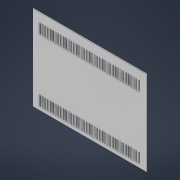
# Autodesk Inventor part: motorRAMM
Saved by Autodesk Inventor 2022 (Build 260153070, 153G)
## iProperties
Created: 2021-12-13
Part Number: motorRAMM
Material: Сталь, окрашенная, слоновая кость, матовая
Document SubType Name: Sheet Metal
Designer: A
Density: 7.85 g/cm^3
Appearance: Гладкая — черная
Mass: 360.681 g
Surface Area: 675.352 cm^2
Volume: 45.9466 cm^3
Sheet Metal Rule: По умолчанию_мм
Author: A
Autodesk Inventor part; units mm, degrees
ref_plane "YZ Plane" through (0, 0, 0) normal (1, 0, 0) x (0, 1, 0)
ref_plane "XZ Plane" through (0, 0, 0) normal (0, 1, 0) x (-1, 0, 0)
ref_plane "XY Plane" through (0, 0, 0) normal (0, 0, 1) x (1, 0, 0)
sketch "Эскиз2" plane through (0, 0, 0) normal (0, 0, 1) x (1, 0, 0)
  line L0 (6, 0) -> (6, 18) construction
  line L1 (7.5, 0) -> (7.5, 18)
  line L2 (4.5, 18) -> (4.5, 0)
  arc A0 (4.5, 0) -> (7.5, 0) centre (6, 0) ccw
  arc A1 (7.5, 18) -> (4.5, 18) centre (6, 18) ccw
  line L3 (210, -7.5) -> (-8, -7.5)
  line L4 (-8, -7.5) -> (-8, 155.5)
  line L5 (-8, 155.5) -> (210, 155.5)
  line L6 (210, 155.5) -> (210, -7.5)
  line L7 (11, 0) -> (11, 18) construction
  line L8 (12.5, 0) -> (12.5, 18)
  line L9 (9.5, 18) -> (9.5, 0)
  arc A2 (9.5, 0) -> (12.5, 0) centre (11, 0) ccw
  arc A3 (12.5, 18) -> (9.5, 18) centre (11, 18) ccw
  line L10 (16, 0) -> (16, 18) construction
  line L11 (17.5, 0) -> (17.5, 18)
  line L12 (14.5, 18) -> (14.5, 0)
  arc A4 (14.5, 0) -> (17.5, 0) centre (16, 0) ccw
  arc A5 (17.5, 18) -> (14.5, 18) centre (16, 18) ccw
  line L13 (21, 0) -> (21, 18) construction
  line L14 (22.5, 0) -> (22.5, 18)
  line L15 (19.5, 18) -> (19.5, 0)
  arc A6 (19.5, 0) -> (22.5, 0) centre (21, 0) ccw
  arc A7 (22.5, 18) -> (19.5, 18) centre (21, 18) ccw
  line L16 (26, 0) -> (26, 18) construction
  line L17 (27.5, 0) -> (27.5, 18)
  line L18 (24.5, 18) -> (24.5, 0)
  arc A8 (24.5, 0) -> (27.5, 0) centre (26, 0) ccw
  arc A9 (27.5, 18) -> (24.5, 18) centre (26, 18) ccw
  line L19 (31, 0) -> (31, 18) construction
  line L20 (32.5, 0) -> (32.5, 18)
  line L21 (29.5, 18) -> (29.5, 0)
  arc A10 (29.5, 0) -> (32.5, 0) centre (31, 0) ccw
  arc A11 (32.5, 18) -> (29.5, 18) centre (31, 18) ccw
  line L22 (36, 0) -> (36, 18) construction
  line L23 (37.5, 0) -> (37.5, 18)
  line L24 (34.5, 18) -> (34.5, 0)
  arc A12 (34.5, 0) -> (37.5, 0) centre (36, 0) ccw
  arc A13 (37.5, 18) -> (34.5, 18) centre (36, 18) ccw
  line L25 (41, 0) -> (41, 18) construction
  line L26 (42.5, 0) -> (42.5, 18)
  line L27 (39.5, 18) -> (39.5, 0)
  arc A14 (39.5, 0) -> (42.5, 0) centre (41, 0) ccw
  arc A15 (42.5, 18) -> (39.5, 18) centre (41, 18) ccw
  line L28 (46, 0) -> (46, 18) construction
  line L29 (47.5, 0) -> (47.5, 18)
  line L30 (44.5, 18) -> (44.5, 0)
  arc A16 (44.5, 0) -> (47.5, 0) centre (46, 0) ccw
  arc A17 (47.5, 18) -> (44.5, 18) centre (46, 18) ccw
  line L31 (51, 0) -> (51, 18) construction
  line L32 (52.5, 0) -> (52.5, 18)
  line L33 (49.5, 18) -> (49.5, 0)
  arc A18 (49.5, 0) -> (52.5, 0) centre (51, 0) ccw
  arc A19 (52.5, 18) -> (49.5, 18) centre (51, 18) ccw
  line L34 (56, 0) -> (56, 18) construction
  line L35 (57.5, 0) -> (57.5, 18)
  line L36 (54.5, 18) -> (54.5, 0)
  arc A20 (54.5, 0) -> (57.5, 0) centre (56, 0) ccw
  arc A21 (57.5, 18) -> (54.5, 18) centre (56, 18) ccw
  line L37 (61, 0) -> (61, 18) construction
  line L38 (62.5, 0) -> (62.5, 18)
  line L39 (59.5, 18) -> (59.5, 0)
  arc A22 (59.5, 0) -> (62.5, 0) centre (61, 0) ccw
  arc A23 (62.5, 18) -> (59.5, 18) centre (61, 18) ccw
  line L40 (66, 0) -> (66, 18) construction
  line L41 (67.5, 0) -> (67.5, 18)
  line L42 (64.5, 18) -> (64.5, 0)
  arc A24 (64.5, 0) -> (67.5, 0) centre (66, 0) ccw
  arc A25 (67.5, 18) -> (64.5, 18) centre (66, 18) ccw
  line L43 (71, 0) -> (71, 18) construction
  line L44 (72.5, 0) -> (72.5, 18)
  line L45 (69.5, 18) -> (69.5, 0)
  arc A26 (69.5, 0) -> (72.5, 0) centre (71, 0) ccw
  arc A27 (72.5, 18) -> (69.5, 18) centre (71, 18) ccw
  line L46 (76, 0) -> (76, 18) construction
  line L47 (77.5, 0) -> (77.5, 18)
  line L48 (74.5, 18) -> (74.5, 0)
  arc A28 (74.5, 0) -> (77.5, 0) centre (76, 0) ccw
  arc A29 (77.5, 18) -> (74.5, 18) centre (76, 18) ccw
  line L49 (81, 0) -> (81, 18) construction
  line L50 (82.5, 0) -> (82.5, 18)
  line L51 (79.5, 18) -> (79.5, 0)
  arc A30 (79.5, 0) -> (82.5, 0) centre (81, 0) ccw
  arc A31 (82.5, 18) -> (79.5, 18) centre (81, 18) ccw
  line L52 (86, 0) -> (86, 18) construction
  line L53 (87.5, 0) -> (87.5, 18)
  line L54 (84.5, 18) -> (84.5, 0)
  arc A32 (84.5, 0) -> (87.5, 0) centre (86, 0) ccw
  arc A33 (87.5, 18) -> (84.5, 18) centre (86, 18) ccw
  line L55 (91, 0) -> (91, 18) construction
  line L56 (92.5, 0) -> (92.5, 18)
  line L57 (89.5, 18) -> (89.5, 0)
  arc A34 (89.5, 0) -> (92.5, 0) centre (91, 0) ccw
  arc A35 (92.5, 18) -> (89.5, 18) centre (91, 18) ccw
  line L58 (96, 0) -> (96, 18) construction
  line L59 (97.5, 0) -> (97.5, 18)
  line L60 (94.5, 18) -> (94.5, 0)
  arc A36 (94.5, 0) -> (97.5, 0) centre (96, 0) ccw
  arc A37 (97.5, 18) -> (94.5, 18) centre (96, 18) ccw
  line L61 (101, 0) -> (101, 18) construction
  line L62 (102.5, 0) -> (102.5, 18)
  line L63 (99.5, 18) -> (99.5, 0)
  arc A38 (99.5, 0) -> (102.5, 0) centre (101, 0) ccw
  arc A39 (102.5, 18) -> (99.5, 18) centre (101, 18) ccw
  line L64 (106, 0) -> (106, 18) construction
  line L65 (107.5, 0) -> (107.5, 18)
  line L66 (104.5, 18) -> (104.5, 0)
  arc A40 (104.5, 0) -> (107.5, 0) centre (106, 0) ccw
  arc A41 (107.5, 18) -> (104.5, 18) centre (106, 18) ccw
  line L67 (111, 0) -> (111, 18) construction
  line L68 (112.5, 0) -> (112.5, 18)
  line L69 (109.5, 18) -> (109.5, 0)
  arc A42 (109.5, 0) -> (112.5, 0) centre (111, 0) ccw
  arc A43 (112.5, 18) -> (109.5, 18) centre (111, 18) ccw
  line L70 (116, 0) -> (116, 18) construction
  line L71 (117.5, 0) -> (117.5, 18)
  line L72 (114.5, 18) -> (114.5, 0)
  arc A44 (114.5, 0) -> (117.5, 0) centre (116, 0) ccw
  arc A45 (117.5, 18) -> (114.5, 18) centre (116, 18) ccw
  line L73 (121, 0) -> (121, 18) construction
  line L74 (122.5, 0) -> (122.5, 18)
  line L75 (119.5, 18) -> (119.5, 0)
  arc A46 (119.5, 0) -> (122.5, 0) centre (121, 0) ccw
  arc A47 (122.5, 18) -> (119.5, 18) centre (121, 18) ccw
  line L76 (126, 0) -> (126, 18) construction
  line L77 (127.5, 0) -> (127.5, 18)
  line L78 (124.5, 18) -> (124.5, 0)
  arc A48 (124.5, 0) -> (127.5, 0) centre (126, 0) ccw
  arc A49 (127.5, 18) -> (124.5, 18) centre (126, 18) ccw
  line L79 (131, 0) -> (131, 18) construction
  line L80 (132.5, 0) -> (132.5, 18)
  line L81 (129.5, 18) -> (129.5, 0)
  arc A50 (129.5, 0) -> (132.5, 0) centre (131, 0) ccw
  arc A51 (132.5, 18) -> (129.5, 18) centre (131, 18) ccw
  line L82 (136, 0) -> (136, 18) construction
  line L83 (137.5, 0) -> (137.5, 18)
  line L84 (134.5, 18) -> (134.5, 0)
  arc A52 (134.5, 0) -> (137.5, 0) centre (136, 0) ccw
  arc A53 (137.5, 18) -> (134.5, 18) centre (136, 18) ccw
  line L85 (141, 0) -> (141, 18) construction
  line L86 (142.5, 0) -> (142.5, 18)
  line L87 (139.5, 18) -> (139.5, 0)
  arc A54 (139.5, 0) -> (142.5, 0) centre (141, 0) ccw
  arc A55 (142.5, 18) -> (139.5, 18) centre (141, 18) ccw
  line L88 (146, 0) -> (146, 18) construction
  line L89 (147.5, 0) -> (147.5, 18)
  line L90 (144.5, 18) -> (144.5, 0)
  arc A56 (144.5, 0) -> (147.5, 0) centre (146, 0) ccw
  arc A57 (147.5, 18) -> (144.5, 18) centre (146, 18) ccw
  line L91 (151, 0) -> (151, 18) construction
  line L92 (152.5, 0) -> (152.5, 18)
  line L93 (149.5, 18) -> (149.5, 0)
  arc A58 (149.5, 0) -> (152.5, 0) centre (151, 0) ccw
  arc A59 (152.5, 18) -> (149.5, 18) centre (151, 18) ccw
  line L94 (156, 0) -> (156, 18) construction
  line L95 (157.5, 0) -> (157.5, 18)
  line L96 (154.5, 18) -> (154.5, 0)
  arc A60 (154.5, 0) -> (157.5, 0) centre (156, 0) ccw
  arc A61 (157.5, 18) -> (154.5, 18) centre (156, 18) ccw
  line L97 (161, 0) -> (161, 18) construction
  line L98 (162.5, 0) -> (162.5, 18)
  line L99 (159.5, 18) -> (159.5, 0)
  arc A62 (159.5, 0) -> (162.5, 0) centre (161, 0) ccw
  arc A63 (162.5, 18) -> (159.5, 18) centre (161, 18) ccw
  line L100 (166, 0) -> (166, 18) construction
  line L101 (167.5, 0) -> (167.5, 18)
  line L102 (164.5, 18) -> (164.5, 0)
  arc A64 (164.5, 0) -> (167.5, 0) centre (166, 0) ccw
  arc A65 (167.5, 18) -> (164.5, 18) centre (166, 18) ccw
  line L103 (171, 0) -> (171, 18) construction
  line L104 (172.5, 0) -> (172.5, 18)
  line L105 (169.5, 18) -> (169.5, 0)
  arc A66 (169.5, 0) -> (172.5, 0) centre (171, 0) ccw
  arc A67 (172.5, 18) -> (169.5, 18) centre (171, 18) ccw
  line L106 (176, 0) -> (176, 18) construction
  line L107 (177.5, 0) -> (177.5, 18)
  line L108 (174.5, 18) -> (174.5, 0)
  arc A68 (174.5, 0) -> (177.5, 0) centre (176, 0) ccw
  arc A69 (177.5, 18) -> (174.5, 18) centre (176, 18) ccw
  line L109 (181, 0) -> (181, 18) construction
  line L110 (182.5, 0) -> (182.5, 18)
  line L111 (179.5, 18) -> (179.5, 0)
  arc A70 (179.5, 0) -> (182.5, 0) centre (181, 0) ccw
  arc A71 (182.5, 18) -> (179.5, 18) centre (181, 18) ccw
  line L112 (186, 0) -> (186, 18) construction
  line L113 (187.5, 0) -> (187.5, 18)
  line L114 (184.5, 18) -> (184.5, 0)
  arc A72 (184.5, 0) -> (187.5, 0) centre (186, 0) ccw
  arc A73 (187.5, 18) -> (184.5, 18) centre (186, 18) ccw
  line L115 (191, 0) -> (191, 18) construction
  line L116 (192.5, 0) -> (192.5, 18)
  line L117 (189.5, 18) -> (189.5, 0)
  arc A74 (189.5, 0) -> (192.5, 0) centre (191, 0) ccw
  arc A75 (192.5, 18) -> (189.5, 18) centre (191, 18) ccw
  line L118 (196, 0) -> (196, 18) construction
  line L119 (197.5, 0) -> (197.5, 18)
  line L120 (194.5, 18) -> (194.5, 0)
  arc A76 (194.5, 0) -> (197.5, 0) centre (196, 0) ccw
  arc A77 (197.5, 18) -> (194.5, 18) centre (196, 18) ccw
  line L121 (6, 120) -> (6, 138) construction
  line L122 (7.5, 120) -> (7.5, 138)
  line L123 (4.5, 138) -> (4.5, 120)
  arc A78 (4.5, 120) -> (7.5, 120) centre (6, 120) ccw
  arc A79 (7.5, 138) -> (4.5, 138) centre (6, 138) ccw
  line L124 (11, 120) -> (11, 138) construction
  line L125 (12.5, 120) -> (12.5, 138)
  line L126 (9.5, 138) -> (9.5, 120)
  arc A80 (9.5, 120) -> (12.5, 120) centre (11, 120) ccw
  arc A81 (12.5, 138) -> (9.5, 138) centre (11, 138) ccw
  line L127 (16, 120) -> (16, 138) construction
  line L128 (17.5, 120) -> (17.5, 138)
  line L129 (14.5, 138) -> (14.5, 120)
  arc A82 (14.5, 120) -> (17.5, 120) centre (16, 120) ccw
  arc A83 (17.5, 138) -> (14.5, 138) centre (16, 138) ccw
  line L130 (21, 120) -> (21, 138) construction
  line L131 (22.5, 120) -> (22.5, 138)
  line L132 (19.5, 138) -> (19.5, 120)
  arc A84 (19.5, 120) -> (22.5, 120) centre (21, 120) ccw
  arc A85 (22.5, 138) -> (19.5, 138) centre (21, 138) ccw
  line L133 (26, 120) -> (26, 138) construction
  line L134 (27.5, 120) -> (27.5, 138)
  line L135 (24.5, 138) -> (24.5, 120)
  arc A86 (24.5, 120) -> (27.5, 120) centre (26, 120) ccw
  arc A87 (27.5, 138) -> (24.5, 138) centre (26, 138) ccw
  line L136 (31, 120) -> (31, 138) construction
  line L137 (32.5, 120) -> (32.5, 138)
  line L138 (29.5, 138) -> (29.5, 120)
  arc A88 (29.5, 120) -> (32.5, 120) centre (31, 120) ccw
  arc A89 (32.5, 138) -> (29.5, 138) centre (31, 138) ccw
  line L139 (36, 120) -> (36, 138) construction
  line L140 (37.5, 120) -> (37.5, 138)
  line L141 (34.5, 138) -> (34.5, 120)
  arc A90 (34.5, 120) -> (37.5, 120) centre (36, 120) ccw
  arc A91 (37.5, 138) -> (34.5, 138) centre (36, 138) ccw
  line L142 (41, 120) -> (41, 138) construction
  line L143 (42.5, 120) -> (42.5, 138)
  line L144 (39.5, 138) -> (39.5, 120)
  arc A92 (39.5, 120) -> (42.5, 120) centre (41, 120) ccw
  arc A93 (42.5, 138) -> (39.5, 138) centre (41, 138) ccw
  line L145 (46, 120) -> (46, 138) construction
  line L146 (47.5, 120) -> (47.5, 138)
  line L147 (44.5, 138) -> (44.5, 120)
  arc A94 (44.5, 120) -> (47.5, 120) centre (46, 120) ccw
  arc A95 (47.5, 138) -> (44.5, 138) centre (46, 138) ccw
  line L148 (51, 120) -> (51, 138) construction
  line L149 (52.5, 120) -> (52.5, 138)
  line L150 (49.5, 138) -> (49.5, 120)
  arc A96 (49.5, 120) -> (52.5, 120) centre (51, 120) ccw
  arc A97 (52.5, 138) -> (49.5, 138) centre (51, 138) ccw
  line L151 (56, 120) -> (56, 138) construction
  line L152 (57.5, 120) -> (57.5, 138)
  line L153 (54.5, 138) -> (54.5, 120)
  arc A98 (54.5, 120) -> (57.5, 120) centre (56, 120) ccw
  arc A99 (57.5, 138) -> (54.5, 138) centre (56, 138) ccw
  line L154 (61, 120) -> (61, 138) construction
  line L155 (62.5, 120) -> (62.5, 138)
  line L156 (59.5, 138) -> (59.5, 120)
  arc A100 (59.5, 120) -> (62.5, 120) centre (61, 120) ccw
  arc A101 (62.5, 138) -> (59.5, 138) centre (61, 138) ccw
  line L157 (66, 120) -> (66, 138) construction
  line L158 (67.5, 120) -> (67.5, 138)
  line L159 (64.5, 138) -> (64.5, 120)
  arc A102 (64.5, 120) -> (67.5, 120) centre (66, 120) ccw
  arc A103 (67.5, 138) -> (64.5, 138) centre (66, 138) ccw
  line L160 (71, 120) -> (71, 138) construction
  line L161 (72.5, 120) -> (72.5, 138)
  line L162 (69.5, 138) -> (69.5, 120)
  arc A104 (69.5, 120) -> (72.5, 120) centre (71, 120) ccw
  arc A105 (72.5, 138) -> (69.5, 138) centre (71, 138) ccw
  line L163 (76, 120) -> (76, 138) construction
  line L164 (77.5, 120) -> (77.5, 138)
  line L165 (74.5, 138) -> (74.5, 120)
  arc A106 (74.5, 120) -> (77.5, 120) centre (76, 120) ccw
  arc A107 (77.5, 138) -> (74.5, 138) centre (76, 138) ccw
  line L166 (81, 120) -> (81, 138) construction
  line L167 (82.5, 120) -> (82.5, 138)
  line L168 (79.5, 138) -> (79.5, 120)
  arc A108 (79.5, 120) -> (82.5, 120) centre (81, 120) ccw
  arc A109 (82.5, 138) -> (79.5, 138) centre (81, 138) ccw
  line L169 (86, 120) -> (86, 138) construction
  line L170 (87.5, 120) -> (87.5, 138)
  line L171 (84.5, 138) -> (84.5, 120)
  arc A110 (84.5, 120) -> (87.5, 120) centre (86, 120) ccw
  arc A111 (87.5, 138) -> (84.5, 138) centre (86, 138) ccw
  line L172 (91, 120) -> (91, 138) construction
  line L173 (92.5, 120) -> (92.5, 138)
  line L174 (89.5, 138) -> (89.5, 120)
  arc A112 (89.5, 120) -> (92.5, 120) centre (91, 120) ccw
  arc A113 (92.5, 138) -> (89.5, 138) centre (91, 138) ccw
  line L175 (96, 120) -> (96, 138) construction
  line L176 (97.5, 120) -> (97.5, 138)
  line L177 (94.5, 138) -> (94.5, 120)
  arc A114 (94.5, 120) -> (97.5, 120) centre (96, 120) ccw
  arc A115 (97.5, 138) -> (94.5, 138) centre (96, 138) ccw
  line L178 (101, 120) -> (101, 138) construction
  line L179 (102.5, 120) -> (102.5, 138)
  line L180 (99.5, 138) -> (99.5, 120)
  arc A116 (99.5, 120) -> (102.5, 120) centre (101, 120) ccw
  arc A117 (102.5, 138) -> (99.5, 138) centre (101, 138) ccw
  line L181 (106, 120) -> (106, 138) construction
  line L182 (107.5, 120) -> (107.5, 138)
  line L183 (104.5, 138) -> (104.5, 120)
  arc A118 (104.5, 120) -> (107.5, 120) centre (106, 120) ccw
  arc A119 (107.5, 138) -> (104.5, 138) centre (106, 138) ccw
  line L184 (111, 120) -> (111, 138) construction
  line L185 (112.5, 120) -> (112.5, 138)
  line L186 (109.5, 138) -> (109.5, 120)
  arc A120 (109.5, 120) -> (112.5, 120) centre (111, 120) ccw
  arc A121 (112.5, 138) -> (109.5, 138) centre (111, 138) ccw
  line L187 (116, 120) -> (116, 138) construction
  line L188 (117.5, 120) -> (117.5, 138)
  line L189 (114.5, 138) -> (114.5, 120)
  arc A122 (114.5, 120) -> (117.5, 120) centre (116, 120) ccw
  arc A123 (117.5, 138) -> (114.5, 138) centre (116, 138) ccw
  line L190 (121, 120) -> (121, 138) construction
  line L191 (122.5, 120) -> (122.5, 138)
  line L192 (119.5, 138) -> (119.5, 120)
  arc A124 (119.5, 120) -> (122.5, 120) centre (121, 120) ccw
  arc A125 (122.5, 138) -> (119.5, 138) centre (121, 138) ccw
  line L193 (126, 120) -> (126, 138) construction
  line L194 (127.5, 120) -> (127.5, 138)
  line L195 (124.5, 138) -> (124.5, 120)
  arc A126 (124.5, 120) -> (127.5, 120) centre (126, 120) ccw
  arc A127 (127.5, 138) -> (124.5, 138) centre (126, 138) ccw
  line L196 (131, 120) -> (131, 138) construction
  line L197 (132.5, 120) -> (132.5, 138)
  line L198 (129.5, 138) -> (129.5, 120)
  arc A128 (129.5, 120) -> (132.5, 120) centre (131, 120) ccw
  arc A129 (132.5, 138) -> (129.5, 138) centre (131, 138) ccw
  line L199 (136, 120) -> (136, 138) construction
  line L200 (137.5, 120) -> (137.5, 138)
  line L201 (134.5, 138) -> (134.5, 120)
  arc A130 (134.5, 120) -> (137.5, 120) centre (136, 120) ccw
  arc A131 (137.5, 138) -> (134.5, 138) centre (136, 138) ccw
  line L202 (141, 120) -> (141, 138) construction
  line L203 (142.5, 120) -> (142.5, 138)
  line L204 (139.5, 138) -> (139.5, 120)
  arc A132 (139.5, 120) -> (142.5, 120) centre (141, 120) ccw
  arc A133 (142.5, 138) -> (139.5, 138) centre (141, 138) ccw
  line L205 (146, 120) -> (146, 138) construction
  line L206 (147.5, 120) -> (147.5, 138)
  line L207 (144.5, 138) -> (144.5, 120)
  arc A134 (144.5, 120) -> (147.5, 120) centre (146, 120) ccw
  arc A135 (147.5, 138) -> (144.5, 138) centre (146, 138) ccw
  line L208 (151, 120) -> (151, 138) construction
  line L209 (152.5, 120) -> (152.5, 138)
  line L210 (149.5, 138) -> (149.5, 120)
  arc A136 (149.5, 120) -> (152.5, 120) centre (151, 120) ccw
  arc A137 (152.5, 138) -> (149.5, 138) centre (151, 138) ccw
  line L211 (156, 120) -> (156, 138) construction
  line L212 (157.5, 120) -> (157.5, 138)
  line L213 (154.5, 138) -> (154.5, 120)
  arc A138 (154.5, 120) -> (157.5, 120) centre (156, 120) ccw
  arc A139 (157.5, 138) -> (154.5, 138) centre (156, 138) ccw
  line L214 (161, 120) -> (161, 138) construction
  line L215 (162.5, 120) -> (162.5, 138)
  line L216 (159.5, 138) -> (159.5, 120)
  arc A140 (159.5, 120) -> (162.5, 120) centre (161, 120) ccw
  arc A141 (162.5, 138) -> (159.5, 138) centre (161, 138) ccw
  line L217 (166, 120) -> (166, 138) construction
  line L218 (167.5, 120) -> (167.5, 138)
  line L219 (164.5, 138) -> (164.5, 120)
  arc A142 (164.5, 120) -> (167.5, 120) centre (166, 120) ccw
  arc A143 (167.5, 138) -> (164.5, 138) centre (166, 138) ccw
  line L220 (171, 120) -> (171, 138) construction
  line L221 (172.5, 120) -> (172.5, 138)
  line L222 (169.5, 138) -> (169.5, 120)
  arc A144 (169.5, 120) -> (172.5, 120) centre (171, 120) ccw
  arc A145 (172.5, 138) -> (169.5, 138) centre (171, 138) ccw
  line L223 (176, 120) -> (176, 138) construction
  line L224 (177.5, 120) -> (177.5, 138)
  line L225 (174.5, 138) -> (174.5, 120)
  arc A146 (174.5, 120) -> (177.5, 120) centre (176, 120) ccw
  arc A147 (177.5, 138) -> (174.5, 138) centre (176, 138) ccw
  line L226 (181, 120) -> (181, 138) construction
  line L227 (182.5, 120) -> (182.5, 138)
  line L228 (179.5, 138) -> (179.5, 120)
  arc A148 (179.5, 120) -> (182.5, 120) centre (181, 120) ccw
  arc A149 (182.5, 138) -> (179.5, 138) centre (181, 138) ccw
  line L229 (186, 120) -> (186, 138) construction
  line L230 (187.5, 120) -> (187.5, 138)
  line L231 (184.5, 138) -> (184.5, 120)
  arc A150 (184.5, 120) -> (187.5, 120) centre (186, 120) ccw
  arc A151 (187.5, 138) -> (184.5, 138) centre (186, 138) ccw
  line L232 (191, 120) -> (191, 138) construction
  line L233 (192.5, 120) -> (192.5, 138)
  line L234 (189.5, 138) -> (189.5, 120)
  arc A152 (189.5, 120) -> (192.5, 120) centre (191, 120) ccw
  arc A153 (192.5, 138) -> (189.5, 138) centre (191, 138) ccw
  line L235 (196, 120) -> (196, 138) construction
  line L236 (197.5, 120) -> (197.5, 138)
  line L237 (194.5, 138) -> (194.5, 120)
  arc A154 (194.5, 120) -> (197.5, 120) centre (196, 120) ccw
  arc A155 (197.5, 138) -> (194.5, 138) centre (196, 138) ccw
  line L238 (196, -1.5) -> (225, -1.5)
  line L239 (196, 19.5) -> (224, 19.5)
  point P0 (6, 9)
  point P1 (11, 9)
  point P2 (16, 9)
  point P3 (21, 9)
  point P4 (26, 9)
  point P5 (31, 9)
  point P6 (36, 9)
  point P7 (41, 9)
  point P8 (46, 9)
  point P9 (51, 9)
  point P10 (56, 9)
  point P11 (61, 9)
  point P12 (66, 9)
  point P13 (71, 9)
  point P14 (76, 9)
  point P15 (81, 9)
  point P16 (86, 9)
  point P17 (91, 9)
  point P18 (96, 9)
  point P19 (101, 9)
  point P20 (106, 9)
  point P21 (111, 9)
  point P22 (116, 9)
  point P23 (121, 9)
  point P24 (126, 9)
  point P25 (131, 9)
  point P26 (136, 9)
  point P27 (141, 9)
  point P28 (146, 9)
  point P29 (151, 9)
  point P30 (156, 9)
  point P31 (161, 9)
  point P32 (166, 9)
  point P33 (171, 9)
  point P34 (176, 9)
  point P35 (181, 9)
  point P36 (186, 9)
  point P37 (191, 9)
  point P38 (196, 9)
  point P39 (6, 129)
  point P40 (11, 129)
  point P41 (16, 129)
  point P42 (21, 129)
  point P43 (26, 129)
  point P44 (31, 129)
  point P45 (36, 129)
  point P46 (41, 129)
  point P47 (46, 129)
  point P48 (51, 129)
  point P49 (56, 129)
  point P50 (61, 129)
  point P51 (66, 129)
  point P52 (71, 129)
  point P53 (76, 129)
  point P54 (81, 129)
  point P55 (86, 129)
  point P56 (91, 129)
  point P57 (96, 129)
  point P58 (101, 129)
  point P59 (106, 129)
  point P60 (111, 129)
  point P61 (116, 129)
  point P62 (121, 129)
  point P63 (126, 129)
  point P64 (131, 129)
  point P65 (136, 129)
  point P66 (141, 129)
  point P67 (146, 129)
  point P68 (151, 129)
  point P69 (156, 129)
  point P70 (161, 129)
  point P71 (166, 129)
  point P72 (171, 129)
  point P73 (176, 129)
  point P74 (181, 129)
  point P75 (186, 129)
  point P76 (191, 129)
  point P77 (196, 129)
  dimension "d13" = 3
  dimension "d14" = 218
  dimension "d15" = 163
  dimension "d18" = 5
  dimension "d21" = 120
  dimension "d26" = 6
  dimension "d27" = 21
  dimension "d28" = 204
  constraints: 636 end point, 314 point on circle, 156 centre point, 4 horizontal, 4 tangent, 3 parallel, 2 vertical, 1 midpoint, 1 perpendicular, 924 other
  measures "d13" diameter of A1
  measures "d14" distance of L4.end L5.end
  measures "d15" distance of L3.end L4.end
  measures "d18" distance of L0.start L7.start
  measures "d21" distance of L0.start L121.start
  measures "d26" distance from line of L3.start L238
  measures "d27" distance between parallel lines of L239 L238
  measures "d28" distance between parallel lines of L6 L0
extrude "Выдавливание2" add sketch "Эскиз2" along normal blind 1.5 contours L3 L4 L5 L6 L239 A77 L120 A76 L238 | L238 A76 L119 A77 L239 L6
chamfer "Фаска1" distance 0.5 angle 45 5 edges at (101, 155.5, 0) (101, 155.5, 1.5) (210, 74, 0) (101, -7.5, 0) (-8, 74, 0)
chamfer "Фаска2" distance 0.5 angle 45 4 edges at (101, 155, 1.5) (210, 73.75, 1.5) (-8, 73.75, 1.5) (101, -7.5, 1.5)
equation "\"Радиус_гибки\" = Толщина"
equation "\"Ширина_просечки\" = Толщина"
equation "\"Глубина_просечки\" = 0.5 * Толщина"
equation "\"Размер_просечки\" = 4 * Толщина"
equation "\"Мин_остаток\" = 2 * Толщина"
equation "\"Радиус_перехода\" = Радиус_гибки"
equation "\"Радиус_Якоби\" = Радиус_гибки"
equation "\"Размер_зазора\" = Толщина"
equation "\"Толщина\" = 1.5"
